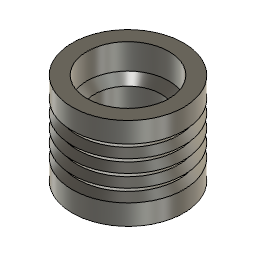
capstan_pulley_ed (Autodesk Fusion 360 design; units mm, degrees)
Autodesk Fusion 360 part; units mm, degrees
sketch "Sketch1" plane through (0, 0, 0) normal (0, 0, 1) x (1, 0, 0)
  circle A0 centre (0, 0) radius 10.936
  dimension "d1" = 21.872
  constraint coincident A0.centre origin
  measures "d1" diameter of A0
extrude "Extrude1" add sketch "Sketch1" along normal mid plane 18
sketch "Sketch2" plane through (0, 0, 9) normal (0, 0, 1) x (-1, 0, 0)
  circle A0 centre (0, 0) radius 10.936
  circle A1 centre (0, 0) radius 8.02
  dimension "d4" = 16.04
  constraint concentric A0 A1
  measures "d4" diameter of A1
extrude "Extrude2" cut sketch "Sketch2" against normal blind 26 contours A1
sketch "Sketch3" plane through (0, 0, 0) normal (0, 1, 0) x (1, 0, 0)
  line L0 (-10.936, -9) -> (10.936, -9) construction
  line L1 (-10.936, 9) -> (10.936, 9) construction
  line L2 (10.936, -9) -> (10.936, 9) construction
  line L3 (10.936, 0) -> (9.936, 1.25)
  line L4 (9.936, 1.25) -> (10.936, 2.5)
  line L5 (10.936, 2.5) -> (10.936, 0)
  point P0 (10.936, 1.25)
  dimension "d7" = 2.5
  dimension "d8" = 1
  constraint coincident L0.end L2.start
  constraint coincident L1.end L2.end
  constraint coincident L2 L3.start
  constraint coincident L2 L4.end
  constraint midpoint L5 P0
  constraint horizontal L3.end P0
  constraint horizontal origin L3.start
  measures "d7" distance of L3.start L4.end
  measures "d8" horizontal distance of L3.end L4.end
revolve "Revolve1" cut sketch "Sketch3" angle 360 about axis through (0, 0, 1.75) along (0, 0, 1)
pattern_linear "R-Pattern1" count 4 spacing 2.5 along (0, 0, 1) both ways of "Revolve1"
ref_plane "WorkPlane1" through (0, 0, 2) normal (0, 0, -1) x (-1, 0, 0)
sketch "Sketch5" plane through (0, 0, 0) normal (0, 1, 0) x (1, 0, 0)
  line L0 (6.52, -2.5) -> (6.52, 2.5)
  line L1 (6.52, -2.5) -> (8.02, -4)
  line L2 (6.52, 2.5) -> (8.02, 4)
  line L3 (8.02, -4) -> (8.02, 4)
  point P0 (8.02, -9)
  point P1 (8.02, 9)
  point P2 (6.52, 0)
  dimension "d18" = 45
  dimension "d19" = 45
  dimension "d20" = 5
  dimension "d21" = 1.5
  constraint vertical L0
  constraint vertical P0 L1.end
  constraint vertical P1 L2.end
  constraint midpoint L0 P2
  constraint horizontal P2 origin
  measures "d18" angle of L0 L2
  measures "d19" angle of L0 L1
  measures "d20" distance of P0 L1.end
  measures "d21" horizontal distance of L0.start L1.end
revolve "Revolve2" add sketch "Sketch5" angle 360 about axis through (0, 0, 1.75) along (0, 0, 1)
equation "d1 = 20.372 mm + 2 * teeth - 0.5 mm"
equation "d8 = teeth"
equation "teeth = 1 mm"
